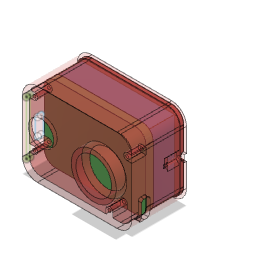
Enclosure (Autodesk Fusion 360 design; units mm, degrees)
Autodesk Fusion 360 part; units mm, degrees
sketch "Board" plane through (0, 0, 0) normal (0, 0, 1) x (1, 0, 0)
  line L0 (4.75, 0) -> (39.105, 0)
  line L1 (43.855, 4.75) -> (43.855, 27.9)
  line L2 (39.105, 32.65) -> (4.75, 32.65)
  line L3 (0, 27.9) -> (0, 4.75)
  arc A0 (4.75, 32.65) -> (0, 27.9) centre (4.75, 27.9) ccw
  arc A1 (43.855, 27.9) -> (39.105, 32.65) centre (39.105, 27.9) ccw
  arc A2 (39.105, 0) -> (43.855, 4.75) centre (39.105, 4.75) ccw
  arc A3 (0, 4.75) -> (4.75, 0) centre (4.75, 4.75) ccw
  line L4 (-0.15, 27.9) -> (-0.15, 4.75)
  arc A4 (-0.15, 4.75) -> (4.75, -0.15) centre (4.75, 4.75) ccw
  line L5 (4.75, -0.15) -> (39.105, -0.15)
  arc A5 (39.105, -0.15) -> (44.005, 4.75) centre (39.105, 4.75) ccw
  line L6 (44.005, 4.75) -> (44.005, 27.9)
  arc A6 (44.005, 27.9) -> (39.105, 32.8) centre (39.105, 27.9) ccw
  line L7 (39.105, 32.8) -> (4.75, 32.8)
  arc A7 (4.75, 32.8) -> (-0.15, 27.9) centre (4.75, 27.9) ccw
  line L8 (-0.35, 27.9) -> (-0.35, 4.75)
  arc A8 (-0.35, 4.75) -> (4.75, -0.35) centre (4.75, 4.75) ccw
  line L9 (4.75, -0.35) -> (39.105, -0.35)
  arc A9 (39.105, -0.35) -> (44.205, 4.75) centre (39.105, 4.75) ccw
  line L10 (44.205, 4.75) -> (44.205, 27.9)
  arc A10 (44.205, 27.9) -> (39.105, 33) centre (39.105, 27.9) ccw
  line L11 (39.105, 33) -> (4.75, 33)
  arc A11 (4.75, 33) -> (-0.35, 27.9) centre (4.75, 27.9) ccw
  line L12 (-0.5, 27.9) -> (-0.5, 4.75)
  arc A12 (-0.5, 4.75) -> (4.75, -0.5) centre (4.75, 4.75) ccw
  line L13 (4.75, -0.5) -> (39.105, -0.5)
  arc A13 (39.105, -0.5) -> (44.355, 4.75) centre (39.105, 4.75) ccw
  line L14 (44.355, 4.75) -> (44.355, 27.9)
  arc A14 (44.355, 27.9) -> (39.105, 33.15) centre (39.105, 27.9) ccw
  line L15 (39.105, 33.15) -> (4.75, 33.15)
  arc A15 (4.75, 33.15) -> (-0.5, 27.9) centre (4.75, 27.9) ccw
  line L16 (21.9275, 32.65) -> (21.9275, 0)
  point P0 (21.9275, 16.325)
  dimension "d329" = 43.855
  dimension "d330" = 32.65
  dimension "d331" = 4.75
  dimension "d332" = 0.15
  dimension "d336" = 0.35
  dimension "d337" = 0.5
  constraint horizontal L0
  constraint vertical L1
  constraint horizontal L2
  constraint vertical L3
  constraint tangent L2 A0
  constraint tangent L3 A0
  constraint tangent L1 A1
  constraint tangent L2 A1
  constraint equal A0 A1
  constraint tangent L0 A2
  constraint tangent L1 A2
  constraint equal A0 A2
  constraint tangent L0 A3
  constraint tangent L3 A3
  constraint equal A0 A3
  constraint midpoint L2 L16.start
  constraint midpoint L0 L16.end
  constraint midpoint L16 P0
  measures "d329" distance of L1 L3
  measures "d330" distance of L0 L2
  measures "d331" radius of A0
sketch "MountPoints" plane through (0, 0, 0) normal (0, 0, 1) x (1, 0, 0)
  line L0 (-0.15, 29.9) -> (0.44, 29.9)
  line L1 (0.44, 29.9) -> (0.44, 26.9)
  line L2 (0.44, 26.9) -> (-0.15, 26.9)
  line L3 (-0.15, 26.9) -> (-0.15, 29.9)
  line L4 (0.44, 29.9) -> (1.94, 29.9)
  line L5 (3.44, 28.4) -> (3.44, 28.4)
  line L6 (1.94, 26.9) -> (0.44, 26.9)
  line L7 (0.44, 26.9) -> (0.44, 29.9)
  line L8 (43.472, 27.333) -> (44.005, 27.333)
  line L9 (44.005, 27.333) -> (44.005, 24.333)
  line L10 (44.005, 24.333) -> (43.472, 24.333)
  line L11 (43.472, 24.333) -> (43.472, 27.333)
  line L12 (41.972, 27.333) -> (43.472, 27.333)
  line L13 (43.472, 27.333) -> (43.472, 24.333)
  line L14 (43.472, 24.333) -> (41.972, 24.333)
  line L15 (40.472, 25.833) -> (40.472, 25.833)
  line L16 (34.3061, 3.4078) -> (34.3065, 3.4078)
  line L17 (35.8063, 1.9078) -> (35.8063, 0.4078)
  line L18 (35.8063, 0.4078) -> (32.8063, 0.4078)
  line L19 (32.8063, 0.4078) -> (32.8063, 1.9078)
  line L20 (32.8063, 0.4078) -> (35.8063, 0.4078)
  line L21 (35.8063, 0.4078) -> (35.8063, -0.15)
  line L22 (35.8063, -0.15) -> (32.8063, -0.15)
  line L23 (32.8063, -0.15) -> (32.8063, 0.4078)
  line L24 (0.39, 9.672) -> (1.89, 9.672)
  line L25 (3.39, 8.172) -> (3.39, 8.172)
  line L26 (1.89, 6.672) -> (0.39, 6.672)
  line L27 (0.39, 6.672) -> (0.39, 9.672)
  line L28 (-0.15, 9.672) -> (0.39, 9.672)
  line L29 (0.39, 9.672) -> (0.39, 6.672)
  line L30 (0.39, 6.672) -> (-0.15, 6.672)
  line L31 (-0.15, 6.672) -> (-0.15, 9.672)
  line L32 (-0.15, 27.9) -> (-0.15, 4.75)
  line L33 (44.005, 4.75) -> (44.005, 27.9)
  line L34 (4.75, -0.15) -> (39.105, -0.15)
  line L35 (0.44, 28.4) -> (3.44, 28.4) construction
  line L36 (40.472, 25.833) -> (43.472, 25.833) construction
  line L37 (32.8063, 1.9078) -> (35.8063, 1.9078) construction
  line L38 (0.39, 8.172) -> (3.39, 8.172) construction
  line L39 (0, 27.9) -> (0, 4.75) construction
  line L40 (4.75, 0) -> (39.105, 0) construction
  arc A0 (3.44, 28.4) -> (1.94, 29.9) centre (1.94, 28.4) ccw
  arc A1 (1.94, 26.9) -> (3.44, 28.4) centre (1.94, 28.4) ccw
  arc A2 (41.972, 27.333) -> (40.472, 25.833) centre (41.972, 25.833) ccw
  arc A3 (40.472, 25.833) -> (41.972, 24.333) centre (41.972, 25.833) ccw
  arc A4 (34.3061, 3.4078) -> (32.8063, 1.9078) centre (34.3063, 1.9078) ccw
  arc A5 (35.8063, 1.9078) -> (34.3065, 3.4078) centre (34.3063, 1.9078) ccw
  arc A6 (3.39, 8.172) -> (1.89, 9.672) centre (1.89, 8.172) ccw
  arc A7 (1.89, 6.672) -> (3.39, 8.172) centre (1.89, 8.172) ccw
  point P0 (1.94, 28.4)
  point P1 (41.972, 25.833)
  point P2 (34.3063, 1.9078)
  point P3 (1.89, 8.172)
  dimension "d404" = 3
  dimension "d407" = 3
  dimension "d409" = 3
  dimension "d411" = 3
  dimension "d412" = 1.89
  dimension "d413" = 8.172
  dimension "d414" = 34.3063
  dimension "d415" = 1.9078
  dimension "d416" = 41.972
  dimension "d417" = 25.833
  dimension "d418" = 1.94
  dimension "d419" = 28.4
  dimension "d422" = 1.5
  constraint horizontal L0
  constraint vertical L1
  constraint horizontal L2
  constraint vertical L3
  constraint horizontal L4
  constraint horizontal L6
  constraint vertical L7
  constraint horizontal L8
  constraint vertical L9
  constraint horizontal L10
  constraint vertical L11
  constraint horizontal L12
  constraint vertical L13
  constraint horizontal L14
  constraint vertical L17
  constraint horizontal L18
  constraint vertical L19
  constraint horizontal L20
  constraint vertical L21
  constraint horizontal L22
  constraint vertical L23
  constraint horizontal L24
  constraint horizontal L26
  constraint vertical L27
  constraint horizontal L28
  constraint vertical L29
  constraint horizontal L30
  constraint vertical L31
  constraint collinear L1 L7
  constraint collinear L0 L4
  constraint collinear L2 L6
  constraint collinear L3 L32
  constraint collinear L11 L13
  constraint collinear L9 L33
  constraint collinear L8 L12
  constraint collinear L10 L14
  constraint collinear L18 L20
  constraint collinear L22 L34
  constraint collinear L19 L23
  constraint collinear L17 L21
  constraint collinear L27 L29
  constraint collinear L24 L28
  constraint collinear L26 L30
  constraint collinear L31 L32
  constraint midpoint L1 L35.start
  constraint midpoint L13 L36.end
  constraint midpoint L29 L38.start
  constraint midpoint L35 P0
  constraint midpoint L36 P1
  constraint midpoint L37 P2
  constraint midpoint L38 P3
  constraint tangent L4 A0
  constraint tangent L6 A1
  constraint equal A0 A1
  constraint tangent L12 A2
  constraint equal A0 A2
  constraint tangent L14 A3
  constraint equal A0 A3
  constraint coincident L19 L37.start
  constraint tangent L19 A4
  constraint equal A0 A4
  constraint coincident L17 L37.end
  constraint tangent L17 A5
  constraint equal A0 A5
  constraint tangent L24 A6
  constraint equal A0 A6
  constraint tangent L26 A7
  constraint equal A0 A7
  measures "d404" distance of L4 L6
  measures "d407" distance of L12 L14
  measures "d409" distance of L17 L19
  measures "d411" distance of L24 L26
  measures "d412" distance of P3 L39
  measures "d413" distance of P3 L40
  measures "d414" distance of P2 L39
  measures "d415" distance of P2 L40
  measures "d416" distance of P1 L39
  measures "d417" distance of P1 L40
  measures "d418" distance of P0 L39
  measures "d419" distance of P0 L40
  measures "d422" radius of A0
sketch "BackplateMountPoint" plane through (0, 0, 0) normal (0, 0, 1) x (1, 0, 0)
  line L0 (1.35, 17.575) -> (-0.15, 19.075)
  line L1 (-0.15, 19.075) -> (-0.15, 13.575)
  line L2 (-0.15, 13.575) -> (1.35, 15.075)
  line L3 (1.35, 15.075) -> (1.35, 17.575)
  line L4 (1.35, 16.325) -> (-0.15, 16.325) construction
  line L5 (-0.15, 27.9) -> (-0.15, 4.75) construction
  point P0 (-0.05, 16.325)
  dimension "d448" = 1.5
  dimension "d449" = 135
  dimension "d450" = 135
  dimension "d451" = 2.5
  dimension "d452" = 0.1
  constraint midpoint L3 L4.start
  constraint midpoint L1 L4.end
  constraint coincident L4 P0
  constraint midpoint L1 L5
  measures "d448" distance of L1 L3
  measures "d449" angle of L0 L3
  measures "d450" angle of L2 L3
  measures "d451" distance of L0.start L2.end
  measures "d452" distance of L1 P0
extrude "Extrude1" add sketch "Board" along normal blind 23.5 thin wall 1.5 on the left open curves L4 A4 L5 A5 L6 A6 L7 A7 makes body 1 in component "Front-Side"
sketch "FrontHoles" plane through (0, 0, 0) normal (0, 0, 1) x (1, 0, 0)
  line L0 (0, 27.9) -> (0, 4.75)
  line L1 (4.75, 0) -> (39.105, 0)
  circle A0 centre (33.5424, 17.392) radius 7.7
  point P0 (6.2926, 17.392)
  point P1 (33.5424, 17.392)
  dimension "d350" = 6.2926
  dimension "d351" = 17.392
  dimension "d352" = 33.5424
  dimension "d353" = 17.392
  dimension "d368" = 15.4
  constraint coincident P1 A0.centre
  measures "d350" distance of P0 L0
  measures "d351" distance of P0 L1
  measures "d352" distance of P1 L0
  measures "d353" distance of P1 L1
  measures "d368" diameter of A0
extrude "Extrude3" add sketch "Board" along normal blind 1.5 separate body contours L0 L2 L3 A0 A3 L16 | L0 L1 L2 A1 A2 L16 | L4 A4 L5 A5 L6 A6 L7 A7 makes body 2 in component "Front-Side"
hole "Hole1" at (6.2926, 17.392, 0) direction (0, 0, 1) diameter 11 depth 12 tip angle 118 bodies 2 in component "Front-Side"
hole "Hole2" at (33.5424, 17.392, 0) direction (0, 0, 1) diameter 15.4 depth 12 tip angle 118 bodies 2 in component "Front-Side"
extrude "Extrude4" add sketch "FrontHoles" along normal blind 6 thin wall 2 outside separate body makes body 3 in component "Front-Side"
copy_body "Body->Comp3" bodies 2 removing the originals makes body 4 in component "Front"
copy_body "CutPasteBodies1" bodies 3 removing the originals makes body 5 in component "Front"
extrude "Extrude2" add sketch "MountPoints" against normal blind 6.2 separate body makes body 6 at (3.0647, 27.4075, -2.0667) makes body 7 at (3.3895, 8.1346, -4.1333) makes body 8 at (41.1898, 27.1129, -4.1333) makes body 9 at (33.8063, -0.15, -4.1333) in component "Front"
hole "Hole1'" at (41.972, 25.833, 0) at (1.94, 28.4, 0) at (1.89, 8.172, 0) at (34.3063, 1.9078, 0) direction (0, 0, -1) diameter 1.3 depth 6.2 tip angle 180 bodies 6 7 8 9 in component "Front"
extrude "Extrude1'" add sketch "Board" along normal blind 1.5 separate body contours L0 L2 L3 A0 A3 L16 | L0 L1 L2 A1 A2 L16 | L4 A4 L5 A5 L6 A6 L7 A7 | L8 A8 L9 A9 L10 A10 L11 A11 makes body 10 in component "Backplate"
extrude "Extrude5" cut sketch "Board" along normal blind 1.5 contours L0 L2 L3 A0 A3 L16 | L0 L1 L2 A1 A2 L16 | L4 A4 L5 A5 L6 A6 L7 A7 | L8 A8 L9 A9 L10 A10 L11 A11 | L12 A12 L13 A13 L14 A14 L15 A15 bodies 1 in component "Front-Side"
sketch "Sketch1" plane through (0, 0, 0) normal (0, 0, 1) x (1, 0, 0) in component "Battery"
  line L0 (20, 15) -> (-20, 15)
  line L1 (-20, 15) -> (-20, -15)
  line L2 (-20, -15) -> (20, -15)
  line L3 (20, -15) -> (20, 15)
  line L4 (20, 15) -> (-20, -15) construction
  dimension "d443" = 40
  dimension "d444" = 30
  constraint horizontal L0
  constraint vertical L1
  constraint horizontal L2
  constraint vertical L3
  constraint midpoint L4 origin
  measures "d443" distance of L1 L3
  measures "d444" distance of L0 L2
extrude "Extrude1''" add sketch "Sketch1" along normal blind 11.2 separate body makes body 11 in component "Battery"
extrude "Extrude7" add sketch "BackplateMountPoint" along normal blind 5 from surface at 1.5 bodies 1 in component "Front-Side"
ref_plane "WorkPlane3" through (21.9275, 16.325, 11.75) normal (1, 0, 0) x (0, 1, 0) in component "Front-Side"
mirror "Mirror2" about plane through (21.9275, 16.325, 11.75) normal (1, 0, 0) of "Extrude7" in component "Front-Side"
sketch "BackplateScrewHeadInset" plane through (0, 0, 0) normal (0, 0, 1) x (1, 0, 0)
  line L0 (0.45, 17.825) -> (-10.05, 17.825)
  line L1 (-10.05, 17.825) -> (-10.05, 14.825)
  line L2 (-10.05, 14.825) -> (0.45, 14.825)
  line L3 (1.45, 15.825) -> (1.45, 16.825)
  line L4 (1.45, 16.325) -> (-10.05, 16.325)
  arc A0 (1.45, 16.825) -> (0.45, 17.825) centre (0.45, 16.825) ccw
  arc A1 (0.45, 14.825) -> (1.45, 15.825) centre (0.45, 15.825) ccw
  point P0 (-0.05, 16.325)
  point P1 (-0.05, 16.325)
  dimension "d461" = 3
  dimension "d462" = 1.5
  dimension "d463" = 1
  dimension "d464" = 10
  constraint horizontal L0
  constraint vertical L1
  constraint horizontal L2
  constraint vertical L3
  constraint midpoint L1 L4.end
  constraint coincident L4 P1
  constraint coincident L3 L4.start
  constraint tangent L0 A0
  constraint tangent L3 A0
  constraint tangent L2 A1
  constraint tangent L3 A1
  constraint equal A0 A1
  constraint coincident P1 P0
  measures "d461" distance of L0 L2
  measures "d462" distance of L3 P1
  measures "d463" radius of A0
  measures "d464" distance of L1 P1
extrude "Extrude8" cut sketch "BackplateScrewHeadInset" along normal blind 1 bodies 1 in component "Front-Side"
extrude "Extrude2'" cut sketch "BackplateScrewHeadInset" along normal blind 1 bodies 10 in component "Backplate"
hole "Hole5" at (-0.05, 16.325, 0) direction (0, 0, 1) diameter 1.3 depth 8.5 tip angle 180 bodies 1 in component "Front-Side"
hole "Hole1''" at (-0.05, 16.325, 0) direction (0, 0, 1) diameter 1.3 depth 8.5 tip angle 180 bodies 10 in component "Backplate"
sketch "HoleSemicircleTool" plane through (0, 0, 0) normal (0, 0, 1) x (1, 0, 0) in component "Backplate"
  line L0 (-2.65, 16.975) -> (-0.05, 16.975)
  line L1 (-0.05, 16.975) -> (-0.05, 15.675)
  line L2 (-0.05, 15.675) -> (-2.65, 15.675)
  line L3 (-2.65, 15.675) -> (-2.65, 16.975)
  point P0 (-0.05, 16.325)
  dimension "d509" = 1.3
  dimension "d510" = 2.6
  constraint horizontal L0
  constraint vertical L1
  constraint horizontal L2
  constraint vertical L3
  constraint midpoint L1 P0
  measures "d509" distance of L0 L2
  measures "d510" distance of L1 L3
extrude "Extrude3'" cut sketch "HoleSemicircleTool" along normal blind 1.5 bodies 10 in component "Backplate"
mirror "Mirror3" about plane through (21.9275, 16.325, 11.75) normal (1, 0, 0) of "Extrude8", "Hole5" in component "Front-Side"
mirror "Mirror1" about plane through (21.9275, 16.325, 11.75) normal (1, 0, 0) of "Extrude2'", "Hole1''", "Extrude3'" in component "Backplate"
extrude "Extrude1'''" add sketch "Board" along normal blind 3.1 separate body contours L0 L2 L3 A0 A3 L16 | L0 L1 L2 A1 A2 L16 makes body 12 in component "Board"
sketch "USBCPlugCutout" plane through (0, 0, 0) normal (1, 0, 0) x (0, 0, -1) in component "Front-Side"
  line L0 (-22, 4.75) -> (-22, 27.9)
  line L1 (-22, 27.9) -> (-23.5, 27.9)
  line L2 (-23.5, 27.9) -> (-23.5, 4.75)
  line L3 (-23.5, 4.75) -> (-22, 4.75)
  line L4 (-18.715, 19.0109) -> (-17.155, 19.0109)
  line L5 (-16.155, 18.0109) -> (-16.155, 10.6709)
  line L6 (-17.155, 9.6709) -> (-18.715, 9.6709)
  line L7 (-19.715, 10.6709) -> (-19.715, 18.0109)
  arc A0 (-18.715, 19.0109) -> (-19.715, 18.0109) centre (-18.715, 18.0109) ccw
  arc A1 (-16.155, 18.0109) -> (-17.155, 19.0109) centre (-17.155, 18.0109) ccw
  arc A2 (-17.155, 9.6709) -> (-16.155, 10.6709) centre (-17.155, 10.6709) ccw
  arc A3 (-19.715, 10.6709) -> (-18.715, 9.6709) centre (-18.715, 10.6709) ccw
  dimension "d492" = 3.56
  dimension "d493" = 9.34
  dimension "d497" = 1
  dimension "d498" = 1
  dimension "d499" = 1
  constraint horizontal L4
  constraint vertical L5
  constraint vertical L7
  constraint tangent L4 A0
  constraint tangent L7 A0
  constraint tangent L4 A1
  constraint tangent L5 A1
  constraint tangent L5 A2
  constraint tangent L6 A2
  constraint tangent L6 A3
  constraint tangent L7 A3
  constraint equal A2 A3
  measures "d492" distance of L5 L7
  measures "d493" distance of L4 L6
  measures "d497" radius of A0
  measures "d498" radius of A1
  measures "d499" radius of A2
extrude "Extrude9" add sketch "USBCPlugCutout" along normal blind 10 separate body contours L4 L5 L6 L7 A0 A1 A2 A3 makes body 13 in component "Front-Side"
ref_plane "WorkPlane5" through (34.3063, 1.6289, 15.7) normal (0, 0, -1) x (-1, 0, 0) in component "Front-Side"
ref_plane "WorkPlane6" through (42.005, 16.325, 22.75) normal (1, 0, 0) x (0, 1, 0) in component "Front-Side"
move_body "Align3" bodies 13 to x (1, 0, 0) y (0, 1, 0) z (0, 0, 1) at (42.005, 0, 0) in component "Front-Side"
move_body "Align4" bodies 13 to x (1, 0, 0) y (0, 1, 0) z (0, 0, 1) at (0, 0, -0.455) in component "Front-Side"
ref_plane "WorkPlane7" through (21.9275, 0, 0) normal (0, -1, 0) x (1, 0, 0) in component "Front-Side"
ref_plane "WorkPlane9" through (21.9275, 5.2535, 0) normal (0, -1, 0) x (1, 0, 0) in component "Front-Side"
move_body "Align5" bodies 13 to x (1, 0, 0) y (0, 1, 0) z (0, 0, 1) at (0, -9.0874, 0) in component "Front-Side"
combine "Combine3" operation cut target body 1 tool bodies 13 in component "Front-Side"
combine "Combine4" operation add target body 1 tool bodies 4 5 6 9 7 8 body 4 seen with x (1, 0, 0) y (0, 1, 0) z (0, 0, 1) at (0, 0, 22) body 5 seen with x (1, 0, 0) y (0, 1, 0) z (0, 0, 1) at (0, 0, 22) body 6 seen with x (1, 0, 0) y (0, 1, 0) z (0, 0, 1) at (0, 0, 22) body 9 seen with x (1, 0, 0) y (0, 1, 0) z (0, 0, 1) at (0, 0, 22) body 7 seen with x (1, 0, 0) y (0, 1, 0) z (0, 0, 1) at (0, 0, 22) body 8 seen with x (1, 0, 0) y (0, 1, 0) z (0, 0, 1) at (0, 0, 22) in component "Front-Side"
component "Front-Side" placed x (1, 0, 0) y (0, 1, 0) z (0, 0, 1) at (0, 0, 0)
component "Backplate" placed x (1, 0, 0) y (0, 1, 0) z (0, 0, 1) at (0, 0, 0)
component "Battery" placed x (1, 0, 0) y (0, 1, 0) z (0, 0, 1) at (21.9275, 16.325, 1.5)
component "Board" placed x (1, 0, 0) y (0, 1, 0) z (0, 0, 1) at (0, 0, 12.7)
component "Front" placed x (1, 0, 0) y (0, 1, 0) z (0, 0, 1) at (0, 0, 22) in component "Front-Side"
equation "BoardHeight = 32.65 mm"
equation "BoardWidth = 43.855 mm"
equation "EnclosureThickness = 1.5 mm"
equation "ImageSensorX = 33.5424 mm"
equation "ImageSensorY = 17.392 mm"
equation "MotionSensorX = 6.2926 mm"
equation "MotionSensorY = 17.392 mm"
equation "LensHoleDiameter = 15.1 mm + 0.2 mm + EnclosureMfgTol"
equation "MotionSensorDiameter = 10.4 mm + 0.5 mm + EnclosureMfgTol"
equation "LensExtrusionThickness = 2 mm"
equation "LensExtrusionDepth = 6 mm"
equation "OuterEdgeRadius = 6 mm"
equation "BoardRadius = 4.75 mm"
equation "MountPoint1X = 1.89 mm"
equation "MountPoint1Y = 8.172 mm"
equation "MountPointDepth = 6 mm + 0.2 mm"
equation "MountPoint2X = 34.3063 mm"
equation "MountPoint2Y = 1.90778125 mm"
equation "MountPoint3X = 41.97198125 mm"
equation "MountPoint3Y = 25.833 mm"
equation "MountPoint4X = 1.94 mm"
equation "MountPoint4Y = 28.4 mm"
equation "BackplateMountPointDepth = 5 mm"
equation "BackplateMountPointWidth = 1.5 mm"
equation "BackplateMountPointChamfer = 1.9 mm"
equation "HoleDiameter = 1.3 mm"
equation "BatteryWidth = 40 mm"
equation "BatteryHeight = 30 mm"
equation "BatteryThickness = 11 mm + 0.2 mm"
equation "BackplateOverlap = 0.2 mm"
equation "BackplateHoleOffset = 0.1 mm"
equation "ScrewHeadDiameter = 3 mm"
equation "ScrewHeadHeight = 1 mm"
equation "BackplateThickness = 1.5 mm"
equation "EnclosureDepth = EnclosureThickness + MountPointDepth + BoardThickness + BatteryThickness + BackplateThickness"
equation "BoardThickness = 3.1 mm"
equation "BoardEnclosureGap = 0.15 mm"
equation "USBCReceptacleCutoutWidth = USBCReceptacleWidth + USBCReceptacleTolerance + 2 * EnclosureMfgTol"
equation "USBCReceptacleCutoutHeight = USBCReceptacleHeight + USBCReceptacleTolerance + 2 * EnclosureMfgTol"
equation "USBCReceptacleCutoutRadius = 2.4 mm / 2 - 0.2 mm"
equation "USBCReceptacleY = 5.25348125 mm"
equation "USBCReceptacleWidth = 3.16 mm"
equation "d329 = BoardWidth"
equation "d330 = BoardHeight"
equation "d331 = BoardRadius"
equation "d332 = BoardEnclosureGap"
equation "d333 = EnclosureThickness"
equation "d334 = EnclosureDepth"
equation "d336 = BoardEnclosureGap + BackplateOverlap"
equation "d337 = BoardEnclosureGap + BackplateOverlap + 0.15 mm"
equation "d350 = MotionSensorX"
equation "d351 = MotionSensorY"
equation "d352 = ImageSensorX"
equation "d353 = ImageSensorY"
equation "d354 = EnclosureThickness"
equation "d363 = MotionSensorDiameter"
equation "d366 = LensHoleDiameter"
equation "d368 = LensHoleDiameter"
equation "d369 = LensExtrusionThickness"
equation "d370 = LensExtrusionDepth"
equation "d372 = EnclosureThickness"
equation "MountPointWidth = 3 mm"
equation "MountPointHeight = 3 mm"
equation "MountPointRadius = 1.5 mm"
equation "d404 = MountPointHeight"
equation "d407 = MountPointHeight"
equation "d409 = MountPointWidth"
equation "d411 = MountPointHeight"
equation "d412 = MountPoint1X"
equation "d413 = MountPoint1Y"
equation "d414 = MountPoint2X"
equation "d415 = MountPoint2Y"
equation "d416 = MountPoint3X"
equation "d417 = MountPoint3Y"
equation "d418 = MountPoint4X"
equation "d419 = MountPoint4Y"
equation "d420 = -MountPointDepth"
equation "d422 = MountPointRadius"
equation "d423 = MountPointDepth"
equation "d424 = HoleDiameter"
equation "d426 = BackplateThickness"
equation "d443 = BatteryWidth"
equation "d444 = BatteryHeight"
equation "d445 = BatteryThickness"
equation "d448 = BackplateMountPointWidth"
equation "d452 = BackplateHoleOffset"
equation "d453 = EnclosureThickness"
equation "d454 = BackplateMountPointDepth"
equation "d461 = ScrewHeadDiameter"
equation "d462 = ScrewHeadDiameter / 2"
equation "d463 = ScrewHeadDiameter / 3"
equation "d465 = ScrewHeadHeight"
equation "d467 = ScrewHeadHeight"
equation "d473 = EnclosureThickness + BackplateMountPointDepth + 2 mm"
equation "d474 = HoleDiameter"
equation "d476 = EnclosureThickness + BackplateMountPointDepth + 2 mm"
equation "d477 = HoleDiameter"
equation "d479 = BoardThickness"
equation "d492 = USBCReceptacleCutoutWidth"
equation "d493 = USBCReceptacleCutoutHeight"
equation "d497 = USBCReceptacleCutoutRadius"
equation "d498 = USBCReceptacleCutoutRadius"
equation "d499 = USBCReceptacleCutoutRadius"
equation "d502 = EnclosureMfgTol"
equation "d505 = -USBCReceptacleY"
equation "USBCReceptacleHeight = 8.94 mm"
equation "USBCReceptacleTolerance = 0.2 mm"
equation "EnclosureMfgTol = 0.1 mm"
equation "d509 = HoleDiameter"
equation "d510 = HoleDiameter * 2"
equation "d511 = BackplateThickness"
named bodies: "Front", "LensExtrusion", "Backplate", "MountPoint4", "MountPoint1", "MountPoint3", "MountPoint2", "USBCPlugCutout"
